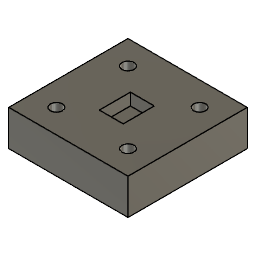
support_axe_y_proto2 (Autodesk Fusion 360 design; units mm, degrees)
Autodesk Fusion 360 part; units mm, degrees
sketch "Esquisse1" plane through (0, 0, 0) normal (0, 0, 1) x (1, 0, 0)
  line L0 (0, 0) -> (50, 0)
  line L1 (50, 0) -> (50, 50)
  line L2 (50, 50) -> (0, 50)
  line L3 (0, 50) -> (0, 0)
  circle A0 centre (10, 40) radius 2.5
  circle A1 centre (40, 40) radius 2.5
  circle A2 centre (10, 10) radius 2.5
  circle A3 centre (40, 10) radius 2.5
  dimension "d1" = 5
  dimension "d2" = 5
  dimension "d3" = 5
  dimension "d4" = 5
  constraint horizontal L0
  constraint vertical L1
  constraint horizontal L2
  constraint vertical L3
  constraint coincident L0.start L3.end
  measures "d1" diameter of A0
  measures "d2" diameter of A1
  measures "d3" diameter of A2
  measures "d4" diameter of A3
extrude "Extrusion1" add sketch "Esquisse1" along normal blind 15
sketch "Esquisse2" plane through (0, 0, 15) normal (0, 0, 1) x (-1, 0, 0)
  circle A0 centre (-10, -40) radius 2.5
  circle A1 centre (-10, -10) radius 2.5
  circle A2 centre (-40, -10) radius 2.5
  circle A3 centre (-40, -40) radius 2.5
  line L0 (0, -50) -> (0, 0)
  line L1 (0, 0) -> (-50, 0)
  line L2 (-50, 0) -> (-50, -50)
  line L3 (-50, -50) -> (0, -50)
  line L4 (0, -25) -> (-20, -25)
  line L5 (-20, -25) -> (-30, -25)
  line L6 (-30, -25) -> (-30, -30)
  line L7 (-30, -30) -> (-20, -30)
  line L8 (-20, -30) -> (-20, -20)
  line L9 (-20, -20) -> (-30, -20)
  line L10 (-30, -20) -> (-30, -25)
  line L11 (-30, -20) -> (-30, -18)
  line L12 (-30, -18) -> (-20, -18)
  line L13 (-20, -18) -> (-20, -20)
  line L14 (-30, -30) -> (-30, -31)
  line L15 (-30, -31) -> (-20, -31)
  line L16 (-20, -31) -> (-20, -30)
  dimension "d7" = 2
  dimension "d8" = 1
  constraint midpoint L0 L4.start
  constraint perpendicular L0 L4
  constraint perpendicular L0 L5
  constraint perpendicular L5 L6
  constraint perpendicular L6 L7
  constraint perpendicular L5 L8
  constraint perpendicular L8 L9
  constraint perpendicular L5 L10
  constraint vertical L11
  constraint perpendicular L11 L12
  constraint perpendicular L9 L13
  constraint vertical L14
  constraint perpendicular L14 L15
  constraint perpendicular L7 L16
  measures "d7" distance of L9.end L11.end
  measures "d8" distance of L6.end L14.end
extrude "Extrusion2" cut sketch "Esquisse2" against normal blind 5 contours L5 L6 L7 L8 | L5 L8 L9 L10 | L7 L14 L15 L16 | L9 L11 L12 L13
